# Autodesk Inventor part: TP
Saved by Autodesk Inventor 2015 SP1 (Build 190203100, 203)
## iProperties
Created: 2015-06-25
Part Number: TP
Material: Generic
Document SubType Name: Modeling
Designer: Patrick
Density: 1 g/cm^3
Appearance: TP_SMALL, TP
Author: Patrick
Autodesk Inventor part; units mm, degrees
ref_plane "YZ Plane" through (0, 0, 0) normal (1, 0, 0) x (0, 1, 0)
ref_plane "XZ Plane" through (0, 0, 0) normal (0, 1, 0) x (-1, 0, 0)
ref_plane "XY Plane" through (0, 0, 0) normal (0, 0, 1) x (1, 0, 0)
sketch "TP_SMALL, TP_253" plane through (0, 0, 0) normal (0, 0, 1) x (1, 0, 0)
  line L0 (-0.5, -0.5) -> (-0.5, 0.5)
  line L1 (-0.5, 0.5) -> (0.5, 0.5)
  line L2 (0.5, 0.5) -> (0.5, -0.5)
  line L3 (0.5, -0.5) -> (-0.5, -0.5)
  constraints: 8 end point
extrude "Extrusion1" add sketch "TP_SMALL, TP_253" along normal blind 1
body "Solid1"
